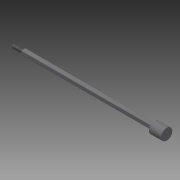
# Autodesk Inventor part: 025.5-D_NR_rod
Saved by Autodesk Inventor 2013 (Build 170138000, 138)
## iProperties
Created: 2013-01-26
Part Number: 025.5-D_NR_rod
Material: Generic
Catalog Web Link: www.cadenas.de
Description: NR_rod-Original Line Cylinders
Vendor: BIMBA
Document SubType Name: Modeling
Designer: actoennies
Manufacturer: BIMBA
Density: 1 g/cm^3
Category: PARTsolutions
Company: BIMBA
Title: 025.5-D_NR_rod
Author: Cadenas PARTsolutions
Comments: Original Line Cylinders
PSOL_IDENT_0: {\\10.0.0.242\data_v9\23d-libs\bimba\bimba\bimba_imperial\bimba_full_line\original_line_cylinders\no
PSOL_IDENT_1: n_rotating_air_cylinders\non_rot_rod.prj},204 {VTYP=3D},{NB=025.5-D_NR_rod},{LINA=025.5-D_NR_rod},{N
PSOL_IDENT_2: N=NR_rod},{DATE=29.09.2011 07:02:13},{GEOMDATE=18.08.2011 05:06:00},{VERSION=},{LINEID=40},{LINESUBI
PSOL_IDENT_3: D=-1},{WBVAR=STROKE,ACTING,MNT,M,NT,EE,EEL,QQ,B}  {NB=025.5-D_NR_rod},{LINA=025.5-D_NR_rod},{KT=DUMM
PSOL_IDENT_4: Y},{PN=025.5-D},{DASH=-},{BORE=0.56250000},{BOREPN=02},{STROKE=5.500},{STROKEALG=[0.001:50/0.001]},{
PSOL_IDENT_5: STROKE1=5.500},{ACTING=D},{ACTINGALG= 'R' , 'Reverse Single Acting' , 'D' , 'Double Acting'  ,'DXDE'
PSOL_IDENT_6: ,'Double Ended Rod'},{ACTINGPN=D},{MNT=},{MNTALG= '' , 'Front Nose Mounting' , 'XP' , 'Double End or
PSOL_IDENT_7: Rear Pivot Mounting' },{TYPE=},{MNTPN=},{NR=},{NRALG= '' , 'N/A' },{NRPN=},{BM=},{BMALG= '' , 'N/A'
PSOL_IDENT_8: },{BMPN=},{CO=},{COALG= '' , 'N/A' },{DER=},{DERALG= '' , 'N/A' },{F=},{FALG= '', 'Standard', 'F',
PSOL_IDENT_9: 'Molycoated Body' },{FPN=},{SR=},{SRALG= '' , '303 Stainless Steel Rod' },{SRPN=},{M=},{MALG= '', 'W
PSOL_IDENT_10: ithout Magnet', 'M', 'With Magnet' },{NT=},{NTPN=},{EE=},{EEL=0},{EEMAX=44.500},{EEALG= '', 'Without
PSOL_IDENT_11: Extra Extension', 'EE', 'With Extra Extension' },{EELALG=0},{EEPN=},{EEPN1=0.000},{G=},{GPN=},{K=},
PSOL_IDENT_12: {KALG= '' , 'N/A' },{KPN=},{Q=},{QQ=},{QALG= '' , 'N/A' },{QPN=},{Y=},{YALG= '' , 'N/A' },{YPN=},{B=
PSOL_IDENT_13: },{BALG= '', 'Without Bumper' , 'B' , 'With Bumper' },{BPN=},{H=},{HALG= '', 'N/A' },{HPN=},{T=},{TA
PSOL_IDENT_14: LG= '' , 'Standard' , 'N' , 'Low Temperature' , 'V' , 'High Temperature' },{NPN=},{VPN=},{W=},{WALG=
PSOL_IDENT_15: '' , 'Without Wiper' , 'W' , 'With Wiper' },{WPN=},{E=},{EALG= '' , 'Without Special Lube and Seals
PSOL_IDENT_16: ' , 'E' , 'With Special Lube and Seals' },{EPN=},{HL=},{HLALG= '' , 'Wihout Low Pressure Hydraulic'
PSOL_IDENT_17: , 'HL' , 'With Low Pressure Hydraulic' },{ST=},{STALG= '' , 'Without Switch Track' , 'T' , 'With Swi
PSOL_IDENT_18: tch Track' },{STP=},{STPALG= '' , 'N/A' },{STPN=},{SER=},{SERALG= '' , 'Without Spring Extend/Return
PSOL_IDENT_19: ' , 'JS' , 'With Spring Return' , 'JR' , 'With Spring Extend' },{PRC=},{PRCALG= '' , 'Without Piston
PSOL_IDENT_20: Rod Clevis' , 'D-166-1' , 'With Piston Rod Clevis' },{PRCPN=},{PB=},{PBALG= '' , 'Without Pivot Bra
PSOL_IDENT_21: cket' , 'D-167' , 'With Pivot Bracket' },{PBPN=},{TLEN=6.3880},{TEXT=0.466667},{SPACE=0.266667},{FRA
PSOL_IDENT_22: C=0.0000},{RGCON=},{RGCON1=},{RGDACCON=R},{RHCON=},{RHCONON=1},{RHACCON=R},{FNUTCON=1},{RNUTCON=0},{
PSOL_IDENT_23: FNUTPN=D-154},{RNUTPN=},{FNUTTRANS=0.0000},{RNUTTRANS=0.0000},{VHOLECON=0},{A1=1.1560},{A1N=1.0310},
PSOL_IDENT_24: {A1P=1.1560},{A1B=0.0000},{A4=0.1570},{A4N=0.5310},{A4P=0.1570},{A5=0.0250},{A1H=0.5},{A1NH=0.5000},
PSOL_IDENT_25: {A1PH=0.9690},{A1BH=0.0000},{A1SH=0.0000},{A2H=0.1570},{A2NH=0.1570},{A2NH1=0.15700000},{A2NH2=0.157
PSOL_IDENT_26: 00000},{LENGTH=2.2800},{LENGTH1=2.2800},{LENGTH2=2.3400},{MUL=5.5000},{MUL11=5.5000},{MUL22=14.4650}
PSOL_IDENT_27: ,{MUL33=8.9650},{MUL2=5.5000},{MUL211=5.5000},{MUL222=2.6300},{MUL233=1.6300},{SSS=11.0000},{RGLEN=1
PSOL_IDENT_28: .0240},{RGLEN1=1.0240},{RHLEN=0.3680},{SSS1=6.0000},{A13=0.7810},{DIF=0.0000},{THDLEN1=0.5000},{THD1
PSOL_IDENT_29: =0.1900},{TAB=UNF},{THDLEN=0.5000},{THD=0.1900},{OD=0.5725},{RODL=7.7800},{PL=0.6240},{RODDIA=0.1870
PSOL_IDENT_30: },{HEX=0.2200},{RODTRANS=0.0000},{G1=0.0000},{ON=0},{G5=0.0000},{DERLEN=7.1560},{THOLE=0.0000},{WF=0
PSOL_IDENT_31: .0000},{WFON=0},{WFL=0.0000},{SSADD=0.0000},{BADD=0.0000},{BADD1=0.125},{MADD=0.0000},{MADD1=0},{BMA
PSOL_IDENT_32: DD1=0.125},{BMADD=0},{NVADD=0.000},{COLOR=0.71,0.71,0.71,0.00},{GROOVE=1},{RL2=0},{RL22=0.5},{RL22NT
PSOL_IDENT_33: =0.5},{RL221=0.5},{RL222X=0},{RL222=0.000},{D1N=0.61500000},{D1B=0.61500000},{D1P=0.00000000},{D1NRH
PSOL_IDENT_34: =0.60950000},{D1PRH=0.61500000},{D1BRH=0.00000000},{D1=0.615},{D1RH=0.6095},{H1=0},{BOZO=0},{CL=0.00
PSOL_IDENT_35: 000000},{WL=0.00000000},{RL=0.00000000},{LXDE=6.65600},{AA=0},{AA1=0.00000000},{AA2=0.00000000},{XDE
PSOL_IDENT_36: DIA=0.19000000},{COR=0.04000000},{EELCP=0}
CNS_NT: Standard
CNS_NB: 025.5-D_NR_rod
CNS_NBSYN: $PN._NR_rod
CNS_LINA: 025.5-D_NR_rod
CNS_PN: 025.5-D
CNS_DASH: -
CNS_BORE: 0.56250000
CNS_BOREPN: 02
CNS_STROKE: 5.500
CNS_STROKEALG: [0.001:50/0.001]
CNS_STROKE1: 5.500
CNS_ACTING: Double Acting
CNS_ACTINGALG: 'R' , 'Reverse Single Acting' , 'D' , 'Double Acting'  ,'DXDE','Double Ended Rod'
CNS_ACTINGPN: D
CNS_MNT: Front Nose Mounting
CNS_MNTALG: '' , 'Front Nose Mounting' , 'XP' , 'Double End or Rear Pivot Mounting'
CNS_NRALG: '' , 'N/A'
CNS_BMALG: '' , 'N/A'
CNS_COALG: '' , 'N/A'
CNS_DERALG: '' , 'N/A'
CNS_FALG: '', 'Standard', 'F', 'Molycoated Body'
CNS_SRALG: '' , '303 Stainless Steel Rod'
CNS_M: Without Magnet
CNS_MALG: '', 'Without Magnet', 'M', 'With Magnet'
CNS_EE: Without Extra Extension
CNS_EEL: 0
CNS_EEMAX: 44.500
CNS_EEALG: '', 'Without Extra Extension', 'EE', 'With Extra Extension'
CNS_EELALG: 0
CNS_EEPN1: 0.000
CNS_KALG: '' , 'N/A'
CNS_QQ: N/A
CNS_QALG: '' , 'N/A'
CNS_YALG: '' , 'N/A'
CNS_B: Without Bumper
CNS_BALG: '', 'Without Bumper' , 'B' , 'With Bumper'
CNS_HALG: '', 'N/A'
CNS_TALG: '' , 'Standard' , 'N' , 'Low Temperature' , 'V' , 'High Temperature'
CNS_WALG: '' , 'Without Wiper' , 'W' , 'With Wiper'
CNS_EALG: '' , 'Without Special Lube and Seals' , 'E' , 'With Special Lube and Seals'
CNS_HLALG: '' , 'Wihout Low Pressure Hydraulic' , 'HL' , 'With Low Pressure Hydraulic'
CNS_STALG: '' , 'Without Switch Track' , 'T' , 'With Switch Track'
CNS_STPALG: '' , 'N/A'
CNS_SERALG: '' , 'Without Spring Extend/Return' , 'JS' , 'With Spring Return' , 'JR' , 'With Spring Extend'
CNS_PRCALG: '' , 'Without Piston Rod Clevis' , 'D-166-1' , 'With Piston Rod Clevis'
CNS_PBALG: '' , 'Without Pivot Bracket' , 'D-167' , 'With Pivot Bracket'
CNS_TLEN: 6.3880
CNS_TEXT: 0.467
CNS_SPACE: 0.267
CNS_FRAC: 0.0000
CNS_RGDACCON: R
CNS_RHCONON: 1
CNS_RHACCON: R
CNS_FNUTCON: 1
CNS_RNUTCON: 0
CNS_FNUTPN: D-154
CNS_FNUTTRANS: 0.0000
CNS_RNUTTRANS: 0.0000
CNS_VHOLECON: 0
CNS_A1: 1.1560
CNS_A1N: 1.0310
CNS_A1P: 1.1560
CNS_A1B: 0.0000
CNS_A4: 0.1570
CNS_A4N: 0.5310
CNS_A4P: 0.1570
CNS_A5: 0.0250
CNS_A1H: 0.500
CNS_A1NH: 0.5000
CNS_A1PH: 0.9690
CNS_A1BH: 0.0000
CNS_A1SH: 0.0000
CNS_A2H: 0.1570
CNS_A2NH: 0.1570
CNS_A2NH1: 0.15700000
CNS_A2NH2: 0.15700000
CNS_LENGTH: 2.2800
CNS_LENGTH1: 2.2800
CNS_LENGTH2: 2.3400
CNS_MUL: 5.5000
CNS_MUL11: 5.5000
CNS_MUL22: 14.4650
CNS_MUL33: 8.9650
CNS_MUL2: 5.5000
CNS_MUL211: 5.5000
CNS_MUL222: 2.6300
CNS_MUL233: 1.6300
CNS_SSS: 11.0000
CNS_RGLEN: 1.0240
CNS_RGLEN1: 1.0240
CNS_RHLEN: 0.3680
CNS_SSS1: 6.0000
CNS_A13: 0.7810
CNS_DIF: 0.0000
CNS_THDLEN1: 0.5000
CNS_THD1: 0.1900
CNS_TAB: UNF
CNS_THDLEN: 0.5000
CNS_THD: 0.1900
CNS_OD: 0.5725
CNS_RODL: 7.7800
CNS_PL: 0.6240
CNS_RODDIA: 0.1870
CNS_HEX: 0.2200
CNS_RODTRANS: 0.0000
CNS_G1: 0.0000
CNS_ON: 0
CNS_G5: 0.0000
CNS_DERLEN: 7.1560
CNS_THOLE: 0.0000
CNS_WF: 0.0000
CNS_WFON: 0
CNS_WFL: 0.0000
CNS_SSADD: 0.0000
CNS_BADD: 0.0000
CNS_BADD1: 0.125
CNS_MADD: 0.0000
CNS_MADD1: 0.000
CNS_BMADD1: 0.125
CNS_BMADD: 0.000
CNS_NVADD: 0.000
CNS_COLOR: 0.71,0.71,0.71,0.00
CNS_GROOVE: 1
CNS_RL2: 0
CNS_RL22: 0.500
CNS_RL22NT: 0.500
CNS_RL221: 0.500
CNS_RL222X: 0.000
CNS_RL222: 0.000
CNS_D1N: 0.61500000
CNS_D1B: 0.61500000
CNS_D1P: 0.00000000
CNS_D1NRH: 0.60950000
CNS_D1PRH: 0.61500000
CNS_D1BRH: 0.00000000
CNS_D1: 0.615
CNS_D1RH: 0.610
CNS_H1: 0.000
CNS_BOZO: 0.000
CNS_CL: 0.00000000
CNS_WL: 0.00000000
CNS_RL: 0.00000000
CNS_LXDE: 6.65600
CNS_AA: 0.000
CNS_AA1: 0.00000000
CNS_AA2: 0.00000000
CNS_XDEDIA: 0.19000000
CNS_COR: 0.04000000
CNS_EELCP: 0.000
SUPPLIER: BIMBA
ARTICLENO: 025.5-D_NR_rod
BOMINFO: 025.5-D_NR_rod
CREATOR: CADENAS GmbH
Autodesk Inventor part; units mm, degrees
ref_plane "YZ Plane" through (0, 0, 0) normal (1, 0, 0) x (0, 1, 0)
ref_plane "XZ Plane" through (0, 0, 0) normal (0, 1, 0) x (-1, 0, 0)
ref_plane "XY Plane" through (0, 0, 0) normal (0, 0, 1) x (1, 0, 0)
sketch "Sketch_1" plane through (0, 0, 0) normal (0, 0, 1) x (1, 0, 0)
  line L0 (184.912, 0) -> (0, 0)
  line L1 (0, 0) -> (0, 2.413)
  arc A0 (1.27, 4.191) -> (0, 2.413) centre (86.3143, -57.8975) ccw
  line L2 (1.27, 4.191) -> (169.0624, 4.191)
  line L3 (169.0624, 4.191) -> (169.0624, 7.22)
  line L4 (169.0624, 7.22) -> (184.912, 7.22)
  line L5 (184.912, 7.22) -> (184.912, 0)
  line L6 (184.912, 0) -> (0, 0)
  constraints: 14 end point, 2 point on circle, 1 centre point
revolve "Revolution1" add sketch "Sketch_1" angle 360 about axis through (184.912, 0, 0) along (1, 0, 0)
sketch "Sketch_3" plane through (0, 0, 0) normal (0, 0, 1) x (1, 0, 0)
  line L0 (0, 0) -> (-12.7, 0)
  line L1 (-12.7, 0) -> (-12.7, 1.9406)
  line L2 (-12.7, 1.9406) -> (-12.2276, 2.413)
  line L3 (-12.2276, 2.413) -> (0, 2.413)
  line L4 (0, 2.413) -> (0, 0)
  line L5 (0, 0) -> (-12.7, 0)
  constraints: 12 end point
revolve "Revolution2" add sketch "Sketch_3" angle 360 about axis through (0, 0, 0) along (1, 0, 0)
thread "Thread1" size "10-32 UNF" class "2A" standard "ANSI Unified Screw Threads" full length
sketch "Sketch_31" plane through (0, 0, 0) normal (1, 0, 0) x (0, 0, -1)
  line L0 (-5.588, 5.588) -> (-5.588, -5.588)
  line L1 (-5.588, -5.588) -> (5.588, -5.588)
  line L2 (5.588, -5.588) -> (5.588, 5.588)
  line L3 (5.588, 5.588) -> (-5.588, 5.588)
  line L4 (-2.794, 1.778) -> (-2.794, -1.778)
  arc A0 (-2.794, -1.778) -> (-1.778, -2.794) centre (-1.778, -1.778) ccw
  line L5 (-1.778, -2.794) -> (1.778, -2.794)
  arc A1 (1.778, -2.794) -> (2.794, -1.778) centre (1.778, -1.778) ccw
  line L6 (2.794, -1.778) -> (2.794, 1.778)
  arc A2 (2.794, 1.778) -> (1.778, 2.794) centre (1.778, 1.778) ccw
  line L7 (1.778, 2.794) -> (-1.778, 2.794)
  arc A3 (-1.778, 2.794) -> (-2.794, 1.778) centre (-1.778, 1.778) ccw
  constraints: 16 end point, 8 point on circle, 4 centre point
extrude "Extrusion1" cut sketch "Sketch_31" along normal mid plane 338.1248
sketch "Sketch_30" plane through (0, 0, 0) normal (0, 0, 1) x (1, 0, 0)
  line L0 (0, 0) -> (-0.254, 0)
  line L1 (-0.254, 2.413) -> (-0.254, 2.159)
  line L2 (-0.254, 2.159) -> (0, 2.159)
  line L3 (0, 2.159) -> (0, 2.413)
  line L4 (0, 2.413) -> (-0.254, 2.413)
  constraints: 10 end point
revolve "Revolution3" cut sketch "Sketch_30" angle 360 about axis through (0, 0, 0) along (1, 0, 0)
ref_plane "rod_cp_XY" through (0, 0, 0) normal (1, 0, 0) x (0, 0, -1)
ref_plane "rod_cp_YZ" through (0, 0, 0) normal (0, 0, -1) x (0, 1, 0)
ref_plane "rod_cp_ZX" through (0, 0, 0) normal (0, 1, 0) x (1, 0, 0)
ref_plane "to_rod_clevis_XY" through (-12.7, 0, 0) normal (1, 0, 0) x (0, 0, -1)
ref_plane "to_rod_clevis_YZ" through (-12.7, 0, 0) normal (0, 0, -1) x (0, 1, 0)
ref_plane "to_rod_clevis_ZX" through (-12.7, 0, 0) normal (0, 1, 0) x (1, 0, 0)
ref_plane "rl22_XY" through (0, 0, 0) normal (1, 0, 0) x (0, 0, -1)
ref_plane "rl22_YZ" through (0, 0, 0) normal (0, 0, -1) x (0, 1, 0)
ref_plane "rl22_ZX" through (0, 0, 0) normal (0, 1, 0) x (1, 0, 0)
ref_plane "rl1_XY" through (-12.7, 0, 0) normal (1, 0, 0) x (0, 0, -1)
ref_plane "rl1_YZ" through (-12.7, 0, 0) normal (0, 0, -1) x (0, 1, 0)
ref_plane "rl1_ZX" through (-12.7, 0, 0) normal (0, 1, 0) x (1, 0, 0)
ref_plane "thd1_XY" through (-12.7, 2.413, 0) normal (1, 0, 0) x (0, 0, -1)
ref_plane "thd1_YZ" through (-12.7, 2.413, 0) normal (0, 0, -1) x (0, 1, 0)
ref_plane "thd1_ZX" through (-12.7, 2.413, 0) normal (0, 1, 0) x (1, 0, 0)
ref_plane "thd2_XY" through (-12.7, -2.413, 0) normal (1, 0, 0) x (0, 0, -1)
ref_plane "thd2_YZ" through (-12.7, -2.413, 0) normal (0, 0, -1) x (0, 1, 0)
ref_plane "thd2_ZX" through (-12.7, -2.413, 0) normal (0, 1, 0) x (1, 0, 0)
ref_plane "dia1_XY" through (0, 2.794, 0) normal (1, 0, 0) x (0, 0, -1)
ref_plane "dia1_YZ" through (0, 2.794, 0) normal (0, 0, -1) x (0, 1, 0)
ref_plane "dia1_ZX" through (0, 2.794, 0) normal (0, 1, 0) x (1, 0, 0)
ref_plane "dia2_XY" through (0, -2.794, 0) normal (1, 0, 0) x (0, 0, -1)
ref_plane "dia2_YZ" through (0, -2.794, 0) normal (0, 0, -1) x (0, 1, 0)
ref_plane "dia2_ZX" through (0, -2.794, 0) normal (0, 1, 0) x (1, 0, 0)
ref_plane "stroke11_XY" through (0, 0, 0) normal (1, 0, 0) x (0, 0, -1)
ref_plane "stroke11_YZ" through (0, 0, 0) normal (0, 0, -1) x (0, 1, 0)
ref_plane "stroke11_ZX" through (0, 0, 0) normal (0, 1, 0) x (1, 0, 0)
ref_plane "h1_XY" through (3.175, 0, 0) normal (0, 0, 1) x (1, 0, 0)
ref_plane "h1_YZ" through (3.175, 0, 0) normal (1, 0, 0) x (0, 1, 0)
ref_plane "h1_ZX" through (3.175, 0, 0) normal (0, 1, 0) x (0, 0, 1)
ref_plane "h2_XY" through (0, 0, 0) normal (0, 0, 1) x (1, 0, 0)
ref_plane "h2_YZ" through (0, 0, 0) normal (1, 0, 0) x (0, 1, 0)
ref_plane "h2_ZX" through (0, 0, 0) normal (0, 1, 0) x (0, 0, 1)
ref_plane "h3_XY" through (0, 0, 0) normal (0, 0, 1) x (1, 0, 0)
ref_plane "h3_YZ" through (0, 0, 0) normal (1, 0, 0) x (0, 1, 0)
ref_plane "h3_ZX" through (0, 0, 0) normal (0, 1, 0) x (0, 0, 1)
ref_plane "rl2_XY" through (0, 0, 0) normal (1, 0, 0) x (0, 0, -1)
ref_plane "rl2_YZ" through (0, 0, 0) normal (0, 0, -1) x (0, 1, 0)
ref_plane "rl2_ZX" through (0, 0, 0) normal (0, 1, 0) x (1, 0, 0)
ref_plane "stroke1_XY" through (0, 0, 0) normal (1, 0, 0) x (0, 0, -1)
ref_plane "stroke1_YZ" through (0, 0, 0) normal (0, 0, -1) x (0, 1, 0)
ref_plane "stroke1_ZX" through (0, 0, 0) normal (0, 1, 0) x (1, 0, 0)
ref_plane "dia12_XY" through (0, 0, 7.8105) normal (1, 0, 0) x (0, 0, -1)
ref_plane "dia12_YZ" through (0, 0, 7.8105) normal (0, 0, -1) x (0, 1, 0)
ref_plane "dia12_ZX" through (0, 0, 7.8105) normal (0, 1, 0) x (1, 0, 0)
ref_plane "dia22_XY" through (0, 0, -7.8105) normal (1, 0, 0) x (0, 0, -1)
ref_plane "dia22_YZ" through (0, 0, -7.8105) normal (0, 0, -1) x (0, 1, 0)
ref_plane "dia22_ZX" through (0, 0, -7.8105) normal (0, 1, 0) x (1, 0, 0)
ref_plane "stroke1bf_XY" through (0, 0, 0) normal (1, 0, 0) x (0, 0, -1)
ref_plane "stroke1bf_YZ" through (0, 0, 0) normal (0, 0, -1) x (0, 1, 0)
ref_plane "stroke1bf_ZX" through (0, 0, 0) normal (0, 1, 0) x (1, 0, 0)
body "Solid1"
